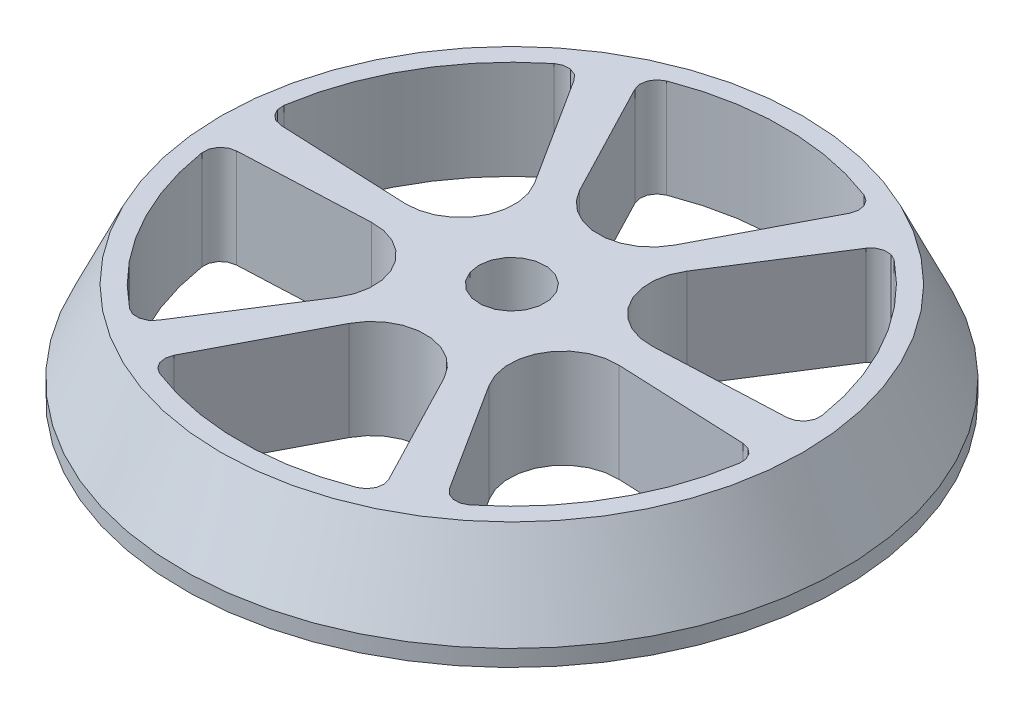
# Autodesk Inventor part: Colossus_7kW_Rotor
Saved by Autodesk Inventor 2014 (Build 180170000, 170)
## iProperties
Created: 2014-11-23
Part Number: Colossus_7kW_Rotor
Material: Générique
Document SubType Name: Modeling
Designer: Yann
Density: 1 g/cm^3
Appearance: Par défaut
Author: Yann
Autodesk Inventor part; units mm, degrees
ref_plane "YZ Plane" through (0, 0, 0) normal (1, 0, 0) x (0, 1, 0)
ref_plane "XZ Plane" through (0, 0, 0) normal (0, 1, 0) x (-1, 0, 0)
ref_plane "XY Plane" through (0, 0, 0) normal (0, 0, 1) x (1, 0, 0)
sketch "Esquisse1" plane through (0, 0, 0) normal (0, 1, 0) x (-1, 0, 0)
  arc A0 (20.5123, 34.3402) -> (-20.5123, 34.3402) centre (0, 0) ccw projected
  circle A1 centre (0, 0) radius 40
  line L0 (0, -56) -> (0, 56) construction
  line L1 (-56, 0) -> (56, 0) construction
  circle A2 centre (0, 0) radius 4
  line L2 (-5.7656, 13.9986) -> (-13.0332, 27.9596)
  line L3 (13.0332, 27.9596) -> (5.7656, 13.9986)
  arc A3 (11.9855, 30.7465) -> (-11.9855, 30.7465) centre (0, 0) ccw
  arc A4 (-5.7656, 13.9986) -> (5.7656, 13.9986) centre (0, 17) ccw
  arc A5 (-11.9855, 30.7465) -> (-13.0332, 27.9596) centre (-11.2592, 28.8831) ccw
  arc A6 (13.0332, 27.9596) -> (11.9855, 30.7465) centre (11.2592, 28.8831) ccw
  line L4 (-15.006, 2.0062) -> (-30.7303, 2.6927)
  line L5 (-17.6971, 25.2668) -> (-9.2404, 11.9924)
  arc A7 (-20.6345, 25.753) -> (-32.62, 4.9935) centre (0, 0) ccw
  arc A8 (-15.006, 2.0062) -> (-9.2404, 11.9924) centre (-14.7224, 8.5) ccw
  arc A9 (-32.62, 4.9935) -> (-30.7303, 2.6927) centre (-30.643, 4.6908) ccw
  arc A10 (-17.6971, 25.2668) -> (-20.6345, 25.753) centre (-19.3839, 24.1922) ccw
  line L6 (-9.2404, -11.9924) -> (-17.6971, -25.2668)
  line L7 (-30.7303, -2.6927) -> (-15.006, -2.0062)
  arc A11 (-32.62, -4.9935) -> (-20.6345, -25.753) centre (0, 0) ccw
  arc A12 (-9.2404, -11.9924) -> (-15.006, -2.0062) centre (-14.7224, -8.5) ccw
  arc A13 (-20.6345, -25.753) -> (-17.6971, -25.2668) centre (-19.3839, -24.1922) ccw
  arc A14 (-30.7303, -2.6927) -> (-32.62, -4.9935) centre (-30.643, -4.6908) ccw
  line L8 (5.7656, -13.9986) -> (13.0332, -27.9596)
  line L9 (-13.0332, -27.9596) -> (-5.7656, -13.9986)
  arc A15 (-11.9855, -30.7465) -> (11.9855, -30.7465) centre (0, 0) ccw
  arc A16 (5.7656, -13.9986) -> (-5.7656, -13.9986) centre (0, -17) ccw
  arc A17 (11.9855, -30.7465) -> (13.0332, -27.9596) centre (11.2592, -28.8831) ccw
  arc A18 (-13.0332, -27.9596) -> (-11.9855, -30.7465) centre (-11.2592, -28.8831) ccw
  line L10 (15.006, -2.0062) -> (30.7303, -2.6927)
  line L11 (17.6971, -25.2668) -> (9.2404, -11.9924)
  arc A19 (20.6345, -25.753) -> (32.62, -4.9935) centre (0, 0) ccw
  arc A20 (15.006, -2.0062) -> (9.2404, -11.9924) centre (14.7224, -8.5) ccw
  arc A21 (32.62, -4.9935) -> (30.7303, -2.6927) centre (30.643, -4.6908) ccw
  arc A22 (17.6971, -25.2668) -> (20.6345, -25.753) centre (19.3839, -24.1922) ccw
  line L12 (9.2404, 11.9924) -> (17.6971, 25.2668)
  line L13 (30.7303, 2.6927) -> (15.006, 2.0062)
  arc A23 (32.62, 4.9935) -> (20.6345, 25.753) centre (0, 0) ccw
  arc A24 (9.2404, 11.9924) -> (15.006, 2.0062) centre (14.7224, 8.5) ccw
  arc A25 (20.6345, 25.753) -> (17.6971, 25.2668) centre (19.3839, 24.1922) ccw
  arc A26 (30.7303, 2.6927) -> (32.62, 4.9935) centre (30.643, 4.6908) ccw
  point P0 (0, 2.9231)
  point P1 (-14.0277, 29.8701)
  point P2 (14.0277, 29.8701)
  point P3 (-2.5315, 1.4615)
  point P4 (-32.8821, 2.7867)
  point P5 (-18.8544, 27.0834)
  point P6 (-2.5315, -1.4615)
  point P7 (-18.8544, -27.0834)
  point P8 (-32.8821, -2.7867)
  point P9 (0, -2.9231)
  point P10 (14.0277, -29.8701)
  point P11 (-14.0277, -29.8701)
  point P12 (2.5315, -1.4615)
  point P13 (32.8821, -2.7867)
  point P14 (18.8544, -27.0834)
  point P15 (2.5315, 1.4615)
  point P16 (18.8544, 27.0834)
  point P17 (32.8821, 2.7867)
  dimension "d0" = 8
  dimension "d1" = 6.5
  dimension "d2" = 2
  dimension "d3" = 7
  dimension "d4" = 17
  dimension "d5" = 55
  dimension "d8" = 360
  constraints: 60 point on circle, 26 centre point, 25 point on line, 24 end point, 6 tangent, 3 coincident, 2 equal radius, 1 symmetric about line, 115 other
  measures "d0" diameter of A2
  measures "d1" radius of A4
  measures "d2" radius of A5
  measures "d3" radial gap between concentric circles of A3 A1
  measures "d4" distance of A4.centre A2.centre
  measures "d5" angle of L3 L2
extrude "Extrusion1" add sketch "Esquisse1" against normal blind 12
chamfer "Chanfrein1" distance 10 angle 25 1 edges at (40, 0, 0) measured on face at (40, -0.5, 0)
